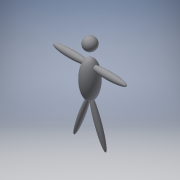
# Autodesk Inventor part: human
Saved by Autodesk Inventor 2019.4 (Build 234330000, 330)
## iProperties
Created: 2019-10-31
Part Number: human
Material: Generic
Document SubType Name: Modeling
Designer: holecep
Density: 1 g/cm^3
Appearance: Default
Author: holecep
Autodesk Inventor part; units mm, degrees
ref_plane "YZ Plane" through (0, 0, 0) normal (1, 0, 0) x (0, 1, 0)
ref_plane "XZ Plane" through (0, 0, 0) normal (0, 1, 0) x (-1, 0, 0)
ref_plane "XY Plane" through (0, 0, 0) normal (0, 0, 1) x (1, 0, 0)
sketch "Sketch1" plane through (0, 0, 0) normal (0, 0, 1) x (1, 0, 0)
  line L0 (0, 0) -> (0, 1905)
  arc A0 (0, 1651) -> (0, 1905) centre (0, 1778) ccw
  ellipse E0 centre (0, 1143) end of major axis (0, 1529.8856) minor radius 173.9104 (0, 756.1144) -> (0, 1529.8856) ccw
  line L1 (0, 1397) -> (-762, 1397)
  line L2 (0, 889) -> (-328.8118, -14.4031)
  ellipse E1 centre (-164.4059, 437.2985) end of major axis (0, 889) minor radius 55.8033 (-328.8118, -14.4031) -> (0, 889) ccw
  ellipse E2 centre (-381, 1397) end of major axis (0, 1397) minor radius 68.7591 (-762, 1397) -> (0, 1397) ccw
  dimension "d0" = 1905
  dimension "d1" = 254
  dimension "d2" = 1143
  dimension "d3" = 1397
  dimension "d4" = 889
  dimension "d5" = 20
  dimension "d6" = 762
  constraints: 4 end point, 2 horizontal, 2 midpoint, 2 point on circle, 1 centre point, 24 other
  measures "d0" distance of A0.end point (0, 0)
  measures "d1" diameter of A0
  measures "d2" distance of point (0, 0) point (0, 1143)
  measures "d3" distance of point (0, 0) L1.start
  measures "d4" distance of L2.start point (0, 0)
  measures "d5" angle to the sketch y axis of L2
  measures "d6" distance of L1.start L1.end
revolve "Revolution1" add sketch "Sketch1" angle 360 about axis through (0, 1397, 0) along (-1, 0, 0) contours E2 L1
revolve "Revolution2" add sketch "Sketch1" angle 360 about axis through (0, 0, 0) along (0, 1, 0) contours E1 L0 | L0 E0 E1
revolve "Revolution3" add sketch "Sketch1" angle 360 about axis through (0, 889, 0) along (-0.3420201, -0.9396926, 0) contours E1 L0 | L0 E1 L2
revolve "Revolution4" add sketch "Sketch1" angle 360 about axis through (0, 0, 0) along (0, 1, 0) contours L0 A0
mirror "Mirror1" about plane through (0, 0, 0) normal (1, 0, 0) of "Revolution1", "Revolution3"
body "Solid1"
